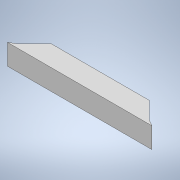
# Autodesk Inventor part: parallel_bar_long_no_hole_v2
Saved by Autodesk Inventor 2022 (Build 260153000, 153)
## iProperties
Created: 2022-06-04
Part Number: parallel_bar_long_no_hole_v2
Material: Generic
Document SubType Name: Modeling
Designer: kylem
Density: 1 g/cm^3
Appearance: Default
Author: kylem
Autodesk Inventor part; units mm, degrees
ref_plane "YZ Plane" through (0, 0, 0) normal (1, 0, 0) x (0, 1, 0)
ref_plane "XZ Plane" through (0, 0, 0) normal (0, 1, 0) x (-1, 0, 0)
ref_plane "XY Plane" through (0, 0, 0) normal (0, 0, 1) x (1, 0, 0)
sketch "Sketch1" plane through (0, 0, 0) normal (0, 1, 0) x (-1, 0, 0)
  line L0 (0, 0) -> (56, 0)
  line L1 (56, 0) -> (54.5, 0)
  line L2 (56, 0) -> (21.359, -20)
  line L3 (56, 0) -> (96, 0) construction
  line L4 (28, 0) -> (28, 5.9969)
  line L5 (0, 0) -> (34.641, -20)
  line L6 (28, 0) -> (28, -8)
  line L7 (28, -8) -> (78, -8)
  line L8 (28, -8) -> (-22, -8)
  line L9 (56, 0) -> (53.4019, -1.5)
  line L10 (53.4019, -1.5) -> (39.2598, -15.6421)
  line L11 (53.4019, -1.5) -> (73.4019, -1.5) construction
  line L12 (2.5981, -1.5) -> (16.7402, -15.6421)
  point P0 (46.9019, -8)
  point P1 (9.0981, -8)
  dimension "d0" = 56
  dimension "d3" = 40
  dimension "d4" = 150
  dimension "d5" = 8
  dimension "d6" = 50
  dimension "d7" = 50
  dimension "d8" = 3
  dimension "d9" = 20
  dimension "d10" = 135
  constraints: 26 end point, 5 horizontal, 3 symmetric about line, 2 equal length, 2 vertical, 1 midpoint, 1 perpendicular, 1 point on line
  measures "d0" distance of L0.start L0.end
  measures "d3" distance of L0.end L2.end
  measures "d4" angle of L2 L3
  measures "d5" distance of L4.start L6.end
  measures "d6" distance of L6.end L7.end
  measures "d7" distance of L6.end L8.end
  measures "d8" distance of L0.end L9.end
  measures "d9" distance of L9.end L10.end
  measures "d10" angle of L10 L11
extrude "Extrusion1" add sketch "Sketch1" along normal blind 8 contours L0 L6 L8 L5 | L0 L2 L7 L6 | L5 L8 L12 | L2 L10 L7
body "Solid1"
